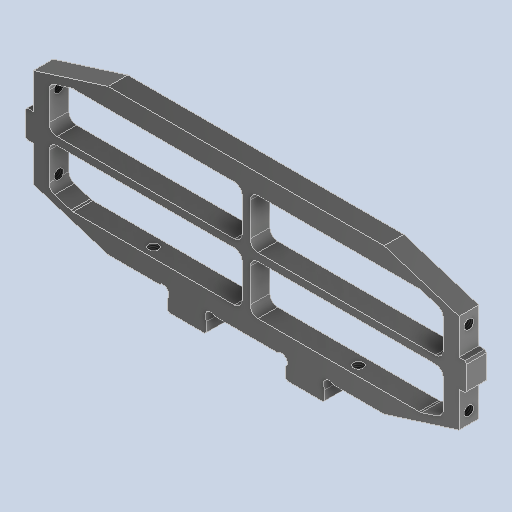
# Autodesk Inventor part: TorsoPelvisBackWallFrame
Saved by Autodesk Inventor 2024.2 (Build 282272000, 272)
## iProperties
Created: 2024-01-26
Part Number: TorsoPelvisBackWallFrame
Material: Acetal Resin, Black
Document SubType Name: Modeling
Designer: Masato Kubotera
Density: 1.425 g/cm^3
Appearance: Smooth - Black
Mass: 10.3269 g
Surface Area: 69.596 cm^2
Volume: 7.24695 cm^3
Vendor: meviy
Author: Masato Kubotera
Autodesk Inventor part; units mm, degrees
ref_plane "YZ Plane" through (0, 0, 0) normal (1, 0, 0) x (0, 1, 0)
ref_plane "XZ Plane" through (0, 0, 0) normal (0, 1, 0) x (-1, 0, 0)
ref_plane "XY Plane" through (0, 0, 0) normal (0, 0, 1) x (1, 0, 0)
sketch "Sketch1" plane through (0, 0, 0) normal (1, 0, 0) x (0, 1, 0)
  line L0 (0, 0) -> (10, 0)
  line L1 (10, 0) -> (10, -5)
  line L2 (10, -5) -> (20, -5)
  line L3 (20, -5) -> (20, 0)
  line L4 (20, 0) -> (54, 0)
  line L5 (54, 0) -> (54, 15)
  line L6 (54, 15) -> (56, 15)
  line L7 (56, 15) -> (56, 22)
  line L8 (56, 22) -> (54, 22)
  line L9 (0, 37) -> (0, 0)
  line L10 (54, 9) -> (50, 9) construction
  line L11 (56, 18.5) -> (54, 18.5) construction
  line L12 (26, 0) -> (26, 5) construction
  line L13 (0, 37) -> (54, 37) construction
  arc A0 (10, -2.1213) -> (7.8787, 0) centre (8.9393, -1.0607) ccw
  line L14 (15, -5) -> (15, 0) construction
  arc A1 (22.1213, 0) -> (20, -2.1213) centre (21.0607, -1.0607) ccw
  line L15 (35, 37) -> (0, 37)
  line L16 (35, 0) -> (54, 6)
  line L17 (35, 37) -> (54, 31)
  line L18 (54, 22) -> (54, 31)
  line L19 (54, 28) -> (50, 28) construction
  line L20 (1, 5) -> (44.1917, 5)
  line L21 (44.1917, 5) -> (50, 6.8342)
  line L22 (50, 6.8342) -> (50, 17.5)
  line L23 (1, 5) -> (1, 17.5)
  line L24 (1, 17.5) -> (50, 17.5)
  line L25 (1, 32) -> (44.1917, 32)
  line L26 (44.1917, 32) -> (50, 30.1658)
  line L27 (50, 30.1658) -> (50, 19.5)
  line L28 (1, 32) -> (1, 19.5)
  line L29 (1, 19.5) -> (50, 19.5)
  point P0 (20, -2.1213)
  point P1 (22.1213, 0)
  dimension "d0" = 5
  dimension "d6" = 2
  dimension "d7" = 4
  dimension "d8" = 6
  dimension "d21" = 3
  dimension "d22" = 70
  dimension "d23" = 10
  dimension "d24" = 5
  dimension "d25" = 6
  dimension "d33" = 37
  dimension "d34" = 1.5
  dimension "d35" = 108
  dimension "d37" = 25
  dimension "d38" = 7
  dimension "d39" = 20
  dimension "d41" = 2
  dimension "d42" = 2
  dimension "d43" = 2
  constraints: 61 end point, 12 point on line, 12 symmetric about line, 10 horizontal, 9 vertical, 5 point on circle, 2 centre point, 2 midpoint, 1 collinear, 1 parallel, 1 perpendicular, 2 other
  measures "d0" distance of L0.end L1.end
  measures "d6" distance of L5.end L6.end
  measures "d7" distance of L10.start L10.end
  measures "d8" distance between parallel lines of L10 L6
  measures "d21" distance of L16.end L10.start
  measures "d22" diameter of L16.start L9
  measures "d23" distance of L1.end L2.end
  measures "d24" distance of L12.start L12.end
  measures "d25" distance between parallel lines of L12 L3
  measures "d33" distance between parallel lines of L0 L13
  measures "d34" radius of A0
  measures "d35" diameter of L18 L9
  measures "d37" distance of L16.end L17.end
  measures "d38" distance of L6.end L7.end
  measures "d39" diameter of L1 L9
  measures "d41" distance between parallel lines of L16 L21
  measures "d42" distance between parallel lines of L24 L29
  measures "d43" diameter of L28 L9
extrude "Extrusion1" add sketch "Sketch1" along normal blind 5 contours L9 L15 L17 L18 L8 L7 L6 L5 L16 L4 A1 L3 L2 L1 A0 L0
sketch "Sketch2" plane through (0, 54, 15) normal (0, 1, 0) x (1, 0, 0)
  line L0 (5, -22) -> (5, 15) projected
  line L1 (5, 6) -> (0, 6)
  line L2 (5, -13) -> (0, -13)
  point P0 (0, 15)
  point P1 (5, -27)
  point P2 (0, 6)
  point P3 (0, 6)
  point P4 (0, 6)
  point P5 (2.5, -13)
  point P6 (2.5, 6)
  constraints: 4 end point, 2 coincident, 2 horizontal, 2 midpoint, 2 point on line
hole "Hole1" at (2.5, 54, 28) at (2.5, 54, 9) direction (0, -1, 0) diameter 2.459 depth 8.8 thread size "M3x0.5" class "6H" standard "ANSI Metric M Profile"
sketch "Sketch3" plane through (0, 20, 0) normal (0, 0, -1) x (-1, 0, 0)
  line L0 (-5, 6) -> (0, 6)
  line L1 (-5, 2.1213) -> (-5, 15) projected
  point P0 (0, -20)
  point P1 (-5, 0)
  point P2 (-2.5, 6)
  point P3 (-5, 34)
  constraints: 2 end point, 1 coincident, 1 horizontal, 1 midpoint, 1 point on line
hole "Hole2" at (2.5, 26, 0) direction (0, 0, 1) diameter 2.459 depth 5 thread size "M3x0.5" class "6H" standard "ANSI Metric M Profile"
fillet "Fillet1" radius 2 10 edges at (2.5, 1, 32) (2.5, 1, 19.5) (2.5, 1, 17.5) (2.5, 1, 5) (2.5, 44.1917, 5) (2.5, 50, 6.8342) (2.5, 50, 17.5) (2.5, 50, 19.5) (2.5, 50, 30.1658) (2.5, 44.1917, 32)
mirror "Mirror3" about plane through (0, 0, 0) normal (0, 1, 0)
chamfer "Chamfer1" distance 0.5 angle 45 8 edges at (2.5, 20, -5) (2.5, 10, -5) (2.5, -10, -5) (2.5, -20, -5) (2.5, -56, 15) (2.5, -56, 22) (2.5, 56, 22) (2.5, 56, 15)
equation "\"d42\" = d41"
equation "\"d31\" = d24"
body "Solid1"
